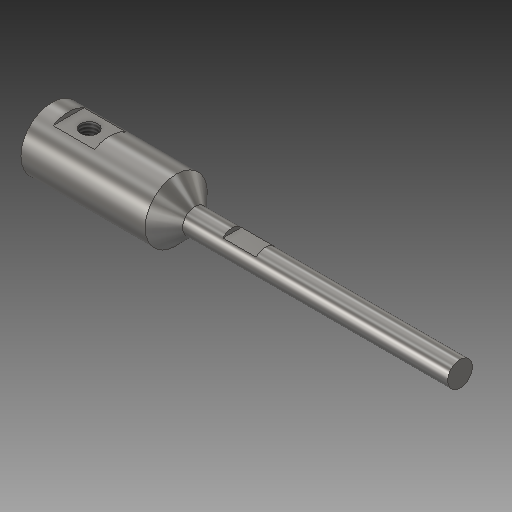
# Autodesk Inventor part: Shaft Kupplung
Saved by Autodesk Inventor 2019 (Build 230136000, 136)
## iProperties
Created: 2021-11-06
Part Number: Shaft Kupplung
Material: Stahl, weich
Document SubType Name: Modeling
Designer: Bergi
Density: 7.85 g/cm^3
Appearance: Halbpoliert
Mass: 49.9896 g
Surface Area: 35.6288 cm^2
Volume: 6.36811 cm^3
Author: Bergi
Autodesk Inventor part; units mm, degrees
note: some values were not read from the file. Chosen so that the rebuilt part matches the saved one: direction of "Bohrung2".
ref_plane "YZ Plane" through (0, 0, 0) normal (1, 0, 0) x (0, 1, 0)
sketch "Skizze1" plane through (0, 0, 0) normal (1, 0, 0) x (0, 1, 0)
  circle A0 centre (0, 0) radius 7.5
  dimension "d0" = 15
  constraints: 1 centre point, 1 coincident
  measures "d0" diameter of A0
extrude "Extrusion1" add sketch "Skizze1" along normal blind 30
sketch "Skizze2" plane through (30, 0, 0) normal (1, 0, 0) x (0, 0, -1)
  circle A0 centre (0, 0) radius 3
  dimension "d3" = 6
  constraints: 1 centre point, 1 coincident
  measures "d3" diameter of A0
extrude "Extrusion2" add sketch "Skizze2" along normal blind 68.5
sketch "Skizze3" plane through (0, 0, 0) normal (-1, 0, 0) x (0, 0, 1)
  circle A0 centre (0, 0) radius 4
  dimension "d6" = 8
  constraints: 1 centre point, 1 coincident
  measures "d6" diameter of A0
hole "Bohrung1" at (0, 0, 0) direction (1, 0, 0) diameter 8 depth 20 tip angle 118
ref_plane "Arbeitsebene1" through (0, 6.5, 0) normal (0, 1, 0) x (-1, 0, 0)
sketch "Skizze4" plane through (0, 6.5, 0) normal (0, 1, 0) x (-1, 0, 0)
  line L0 (-30, 7.5) -> (-30, -7.5) projected
  line L1 (0, -7.5) -> (0, 7.5) projected
  line L2 (0, 7.5) -> (-30, 7.5) projected
  line L3 (0, -7.5) -> (-30, -7.5) projected
  line L4 (-4, -7.5) -> (-4, 7.5)
  line L5 (-14, -7.5) -> (-14, 7.5)
  point P0 (0, 0)
  dimension "d15" = 10
  dimension "d16" = 4
  constraints: 4 end point, 4 point on line, 2 perpendicular
  measures "d15" distance between parallel lines of L5 L4
  measures "d16" distance between parallel lines of L1 L4
extrude "Extrusion3" cut sketch "Skizze4" along normal through all contours L2 L4 L3 L5
sketch "Skizze5" plane through (0, 6.5, 0) normal (0, 1, 0) x (1, 0, 0)
  line L0 (14, -3.7417) -> (4, -3.7417) projected
  line L1 (14, -3.7417) -> (14, 3.7417) projected
  line L2 (4, 3.7417) -> (14, 3.7417) projected
  line L3 (4, 3.7417) -> (4, -3.7417) projected
  line L4 (4, 3.7417) -> (14, -3.7417)
  line L5 (4, 3.7417) -> (14, 3.7417) projected
  line L6 (14, -3.7417) -> (4, -3.7417) projected
  line L7 (14, 3.7417) -> (4, -3.7417)
  point P0 (0, 0)
  point P1 (9, 0)
  constraints: 4 end point, 1 midpoint
hole "Bohrung2" at (9, 6.5, 0) direction (0, -1, 0) diameter 4.134 end up to surface thread size "M5x0.8" class "6H" standard "ISO Metric profile"
chamfer "Fase1" distance 4.5 angle 45 1 edges at (30, 0, 3)
ref_plane "Arbeitsebene2" through (0, 3, 0) normal (0, 1, 0) x (-1, 0, 0)
sketch "Skizze6" plane through (0, 3, 0) normal (0, 1, 0) x (-1, 0, 0)
  line L0 (-118.2, 0) -> (19.7, 0) construction
  line L1 (-43.5, 5) -> (-51.5, 5)
  line L2 (-51.5, 5) -> (-51.5, -5)
  line L3 (-51.5, -5) -> (-43.5, -5)
  line L4 (-43.5, -5) -> (-43.5, 5)
  line L5 (-43.5, 5) -> (-51.5, -5) construction
  line L6 (-51.5, 5) -> (-43.5, -5) construction
  point P0 (0, 0)
  point P1 (-47.5, 0)
  dimension "d30" = 8
  dimension "d31" = 10
  dimension "d32" = 47.5
  constraints: 12 end point, 2 midpoint, 2 parallel, 1 horizontal, 1 perpendicular, 1 point on line
  measures "d30" distance of L3.end L2.end
  measures "d31" distance of L2.end L1.end
  measures "d32" distance of point (-47.5, 0) point (0, 0)
extrude "Extrusion4" cut sketch "Skizze6" against normal blind 1
